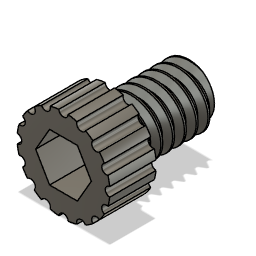
Adjustable Calibrator Base (Autodesk Fusion 360 archive; units mm, degrees)
design "Adjustment Screw"
Autodesk Fusion 360 part; units mm, degrees
sketch "Sketch4" plane through (0, 0, 0) normal (0, 0, 1) x (1, 0, 0)
  circle A0 centre (0, 0) radius 3.175
  dimension "d24" = 6.35
  constraint coincident A0.centre origin
  measures "d24" diameter of A0
extrude "Extrude6" add sketch "Sketch4" along normal blind 8.5
sketch "Sketch5" plane through (0, 0, 0) normal (0, 1, 0) x (1, 0, 0)
  circle A0 centre (0, -3) radius 0.7
  line L0 (-3.175, 0) -> (3.175, 0)
  dimension "d29" = 1.4
  measures "d29" diameter of A0
sketch "Sketch6" plane through (0, 0, 8.5) normal (0, 0, 1) x (1, 0, 0)
  circle A0 centre (0, 0) radius 3.175
  circle A1 centre (0, 0) radius 4
  circle A2 centre (0, 0) radius 3
  dimension "d35" = 8
  dimension "d39" = 6
  constraint coincident A0.centre A1.centre
  measures "d35" diameter of A1
  measures "d39" diameter of A2
sketch "Sketch7" plane through (0, 0, 8.5) normal (0, 0, 1) x (1, 0, 0)
  circle A0 centre (0, 0) radius 3.175
  circle A1 centre (0, 0) radius 5
  constraint coincident A0.centre A1.centre
extrude "Extrude9" add sketch "Sketch7" along normal blind 5 contours A0 | A1
sketch "Sketch8" plane through (0, 0, 13.5) normal (0, 0, 1) x (1, 0, 0)
  circle A0 centre (0, 0) radius 3
  line L0 (0, 0) -> (-3, 0)
  line L1 (0, 0) -> (3, 0)
  line L2 (0, 0) -> (3, 0) construction
  line L3 (0, 0) -> (-1.5, -2.5981)
  line L4 (0, 0) -> (1.5, -2.5981)
  line L5 (0, 0) -> (-1.5, 2.5981)
  line L6 (0, 0) -> (1.5, 2.5981)
  line L7 (-1.5, 2.5981) -> (-3, 0)
  line L8 (-1.5, 2.5981) -> (1.5, 2.5981)
  line L9 (1.5, 2.5981) -> (3, 0)
  line L10 (3, 0) -> (1.5, -2.5981)
  line L11 (1.5, -2.5981) -> (-1.5, -2.5981)
  line L12 (-1.5, -2.5981) -> (-3, 0)
  circle A1 centre (0, 0) radius 5
  dimension "d47" = 60
  dimension "d48" = 60
  dimension "d49" = 60
  constraint coincident A0.centre L0.start
  constraint coincident A0 L0.end
  constraint horizontal L0
  constraint coincident A0 L1.end
  constraint parallel L0 L1
  constraint horizontal L2
  constraint coincident A0 L3.end
  constraint coincident A0 L4.end
  constraint coincident A0 L5.end
  constraint coincident A0 L6.end
  constraint parallel L3 L6
  constraint parallel L9 L12
  measures "d47" angle of L0 L3
  measures "d48" angle of L3 L4
  measures "d49" angle of L0 L5
extrude "Extrude10" cut sketch "Sketch8" against normal blind 4 contours L1 L4 L10 | L1 L6 L9 | L5 L6 L8 | L3 L4 L11 | L0 L3 L12 | L0 L5 L7
sketch "Sketch9" plane through (0, 0, 13.5) normal (0, 0, 1) x (1, 0, 0)
  line L0 (-1.5, -2.5981) -> (-3, 0)
  line L1 (-3, 0) -> (-1.5, 2.5981)
  line L2 (-1.5, 2.5981) -> (1.5, 2.5981)
  line L3 (1.5, 2.5981) -> (3, 0)
  line L4 (3, 0) -> (1.5, -2.5981)
  line L5 (1.5, -2.5981) -> (-1.5, -2.5981)
  circle A0 centre (0, 0) radius 5
  circle A1 centre (0, 5) radius 0.5
  circle A2 centre (-1.9134, 4.6194) radius 0.5
  circle A3 centre (-3.5355, 3.5355) radius 0.5
  circle A4 centre (-4.6194, 1.9134) radius 0.5
  circle A5 centre (-5, 0) radius 0.5
  circle A6 centre (-4.6194, -1.9134) radius 0.5
  circle A7 centre (-3.5355, -3.5355) radius 0.5
  circle A8 centre (-1.9134, -4.6194) radius 0.5
  circle A9 centre (0, -5) radius 0.5
  circle A10 centre (1.9134, -4.6194) radius 0.5
  circle A11 centre (3.5355, -3.5355) radius 0.5
  circle A12 centre (4.6194, -1.9134) radius 0.5
  circle A13 centre (5, 0) radius 0.5
  circle A14 centre (4.6194, 1.9134) radius 0.5
  circle A15 centre (3.5355, 3.5355) radius 0.5
  circle A16 centre (1.9134, 4.6194) radius 0.5
  dimension "d53" = 360
  constraint coincident A0 A1.centre
extrude "Extrude11" cut sketch "Sketch9" against normal blind 5 contours A0 A13 | A0 A14 | A0 A12 | A0 A15 | A0 A11 | A0 A16 | A0 A10 | A0 A1 | A0 A9 | A0 A2 | A0 A8 | A0 A3 | A0 A7 | A0 A4 | A0 A6 | A0 A5 picked at (4.8432, -0.1146) picked at (4.4687, 1.838) picked at (4.4687, -1.838) picked at (3.4082, 3.4252) picked at (3.4082, -3.4252) picked at (1.8602, 4.4595) picked at (1.8602, -4.4595) picked at (-0.0121, 4.8319) picked at (-0.0121, -4.8319) picked at (-1.8522, 4.4624) picked at (-1.8522, -4.4624) picked at (-3.409, 3.4242) picked at (-3.409, -3.4242) picked at (-4.467, 1.8415) picked at (-4.467, -1.8415) picked at (-4.8315, 0)
fillet "Fillet6" radius 0.5 1 edges at (-2.9601, -1.1481, 8.5)
thread "Thread2" "ANSI Unified Screw Threads 0.25 1/4-20 UNC 3A" major diameter 6.2484 minor diameter 4.8387 pitch 1.27 angle 60 modelled right hand crest width 0.1965 on face at (3.1711, -0.1583, 5.3333) crest through (3.1242, 0, -0.3175)
